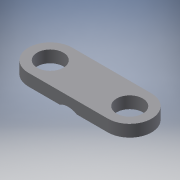
# Autodesk Inventor part: TubeClamp
Saved by Autodesk Inventor 2016 (Build 200138000, 138)
## iProperties
Created: 2015-12-24
Part Number: TubeClamp
Material: Generic
Document SubType Name: Modeling
Designer: inornate
Density: 1 g/cm^3
Appearance: Default
Author: inornate
Autodesk Inventor part; units mm, degrees
ref_plane "YZ Plane" through (0, 0, 0) normal (1, 0, 0) x (0, 1, 0)
ref_plane "XZ Plane" through (0, 0, 0) normal (0, 1, 0) x (-1, 0, 0)
ref_plane "XY Plane" through (0, 0, 0) normal (0, 0, 1) x (1, 0, 0)
sketch "Sketch1" plane through (0, 0, 0) normal (0, 0, 1) x (1, 0, 0)
  circle A0 centre (5.0002, 0) radius 1.25 construction
  line L0 (1.4779, -3) -> (1.4779, 3) construction
  line L1 (5.0002, -3) -> (1.4779, -3) construction
  arc A1 (5.0002, -3) -> (5.0002, 3) centre (5.0002, 0) ccw construction
  line L2 (1.4779, 3) -> (5.0002, 3) construction
  circle A2 centre (-5.0002, 0) radius 1.25 construction
  line L3 (-1.4614, 3) -> (-1.4614, -3) construction
  line L4 (-5.0002, 3) -> (-1.4614, 3) construction
  arc A3 (-5.0002, 3) -> (-5.0002, -3) centre (-5.0002, 0) ccw construction
  line L5 (-1.4614, -3) -> (-5.0002, -3) construction
  line L6 (-5.0002, 0) -> (5.0002, 0) construction
  line L7 (-5.0002, -2.75) -> (5.0002, -2.75)
  line L8 (5.0002, 2.75) -> (-5.0002, 2.75)
  arc A4 (-5.0002, 2.75) -> (-5.0002, -2.75) centre (-5.0002, 0) ccw
  arc A5 (5.0002, -2.75) -> (5.0002, 2.75) centre (5.0002, 0) ccw
  circle A6 centre (-5.0002, 0) radius 1.65
  circle A7 centre (5.0002, 0) radius 1.65
  point P0 (0, 0)
  point P1 (0, 0)
  dimension "d0" = 5.5
  dimension "d1" = 3.3
  dimension "d2" = 3.3
  constraints: 8 end point, 4 centre point, 4 point on circle, 4 tangent, 2 coincident, 2 parallel, 1 midpoint
  measures "d0" diameter of A5
  measures "d1" diameter of A6
  measures "d2" diameter of A7
extrude "Extrusion1" add sketch "Sketch1" along normal blind 1.5
sketch "Sketch2" plane through (-5.0002, 2.75, 0) normal (0, 1, 0) x (1, 0, 0)
  circle A0 centre (5.0085, 1.8) radius 2.1
  arc A1 (5.0085, 3.6) -> (5.0085, -0.6) centre (5.0085, 1.5) ccw projected
  point P0 (5.0002, 0)
  constraints: 1 centre point, 1 equal radius
extrude "Extrusion2" cut sketch "Sketch2" against normal through all
body "Solid1"
